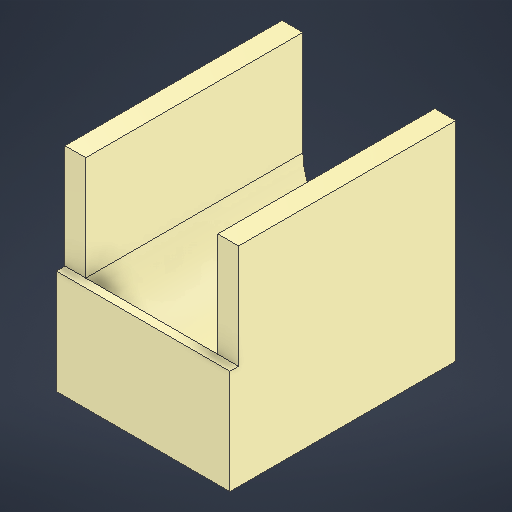
# Autodesk Inventor part: NiMH_Holder_Back
Saved by Autodesk Inventor 2026 (Build 300175050, 175E)
## iProperties
Created: 2025-06-11
Part Number: NiMH_Holder_Back
Material: Generic
Document SubType Name: Modeling
Designer: satom
Density: 1 g/cm^3
Appearance: Default
Author: satom
Autodesk Inventor part; units mm, degrees
ref_plane "YZ Plane" through (0, 0, 0) normal (1, 0, 0) x (0, 1, 0)
ref_plane "XZ Plane" through (0, 0, 0) normal (0, 1, 0) x (-1, 0, 0)
ref_plane "XY Plane" through (0, 0, 0) normal (0, 0, 1) x (1, 0, 0)
sketch "Sketch1" plane through (0, 0, 0) normal (0, 0, 1) x (1, 0, 0)
  line L0 (-15.875, 0) -> (15.875, 0)
  line L1 (15.875, 0) -> (15.875, 38.1)
  line L2 (15.875, 38.1) -> (-15.875, 38.1)
  line L3 (-15.875, 38.1) -> (-15.875, 0)
  point P0 (0, 0)
  dimension "d2" = 31.75
  dimension "d3" = 38.1
  dimension "d4" = 15.875
  dimension "d5" = 0
  constraints: 8 end point, 2 parallel, 1 horizontal, 1 perpendicular
  measures "d2" distance of L0.start L0.end
  measures "d3" distance of L0.end L1.end
  measures "d4" distance from line of point (0, 0) L3
  measures "d5" distance from line of point (0, 0) L0
extrude "Extrusion1" add sketch "Sketch1" along normal blind 139.7
sketch "Sketch2" plane through (0, 0, 139.7) normal (0, 0, 1) x (1, 0, 0)
  arc A0 (-12.065, 19.05) -> (12.065, 19.05) centre (0, 19.05) ccw
  line L0 (-15.875, 0) -> (15.875, 0) projected
  line L1 (12.065, 19.05) -> (12.065, 38.1)
  line L2 (15.875, 38.1) -> (-15.875, 38.1) projected
  line L3 (-12.065, 19.05) -> (-12.065, 38.1)
  point P0 (0, 0)
  dimension "d8" = 19.05
  dimension "d9" = 24.13
  constraints: 4 end point, 2 point on circle, 2 point on line, 1 centre point, 1 parallel, 1 tangent, 1 vertical
  measures "d8" distance from line of L0 A0.centre
  measures "d9" diameter of A0
extrude "Extrusion2" cut sketch "Sketch2" against normal through all
sketch "Sketch3" plane through (-15.875, 0, 0) normal (0, -1, 0) x (1, 0, 0)
  circle A0 centre (28.575, 8.89) radius 2
  circle A1 centre (3.175, 130.81) radius 2
  line L0 (15.875, 0) -> (15.875, 139.7) construction
  line L1 (0, 139.7) -> (31.75, 139.7) construction
  line L2 (0, 0) -> (31.75, 0) construction
  line L3 (31.75, 139.7) -> (0, 139.7) construction
  circle A2 centre (28.575, 111.76) radius 2
  line L4 (31.75, 0) -> (31.75, 139.7) projected
  dimension "d12" = 4
  dimension "d13" = 4
  dimension "d14" = 12.7
  dimension "d15" = 8.89
  dimension "d16" = 12.7
  dimension "d17" = 8.89
  dimension "d28" = 4
  dimension "d30" = 27.94
  dimension "d32" = 12.7
  constraints: 4 end point, 3 centre point, 2 midpoint, 1 collinear
  measures "d12" diameter of A0
  measures "d13" diameter of A1
  measures "d14" distance from line of L0 A0.centre
  measures "d15" distance from line of L2 A0.centre
  measures "d16" distance from line of L0 A1.centre
  measures "d17" vertical distance of L1.start A1.centre
  measures "d28" diameter of A2
  measures "d30" vertical distance of point (15.875, 139.7) A2.centre
  measures "d32" distance from line of A2.centre L0
extrude "Heat Set Inserts" cut sketch "Sketch3" against normal blind 7
sketch "Sketch4" plane through (0, 0, 139.7) normal (0, 0, 1) x (1, 0, 0)
  line L0 (-15.875, 0) -> (15.875, 0) projected
  line L1 (15.875, 0) -> (15.875, 38.1) projected
  line L2 (-15.875, 0) -> (15.875, 0)
  line L3 (15.875, 0) -> (15.875, 19.05)
  line L4 (15.875, 19.05) -> (-15.875, 19.05)
  line L5 (-15.875, 19.05) -> (-15.875, 0)
  point P0 (0, 0)
  dimension "d20" = 19.05
  constraints: 8 end point, 2 parallel, 1 horizontal, 1 midpoint, 1 perpendicular
  measures "d20" distance of L4.end L0.start
extrude "Back Wall" add sketch "Sketch4" along normal blind 1.5875
sketch "Sketch5" plane through (0, 0, 0) normal (0, 0, -1) x (-1, 0, 0)
  line L0 (15.875, 0) -> (-15.875, 0) projected
  line L1 (15.875, 19.05) -> (15.875, 0) projected
  line L2 (-15.875, 0) -> (15.875, 0)
  line L3 (15.875, 0) -> (15.875, 10.16)
  line L4 (15.875, 10.16) -> (-15.875, 10.16)
  line L5 (-15.875, 10.16) -> (-15.875, 0)
  point P0 (0, 0)
  dimension "d23" = 10.16
  constraints: 8 end point, 2 parallel, 1 horizontal, 1 perpendicular, 1 point on line
  measures "d23" distance of L4.end L0.end
extrude "Extrusion5" add sketch "Sketch5" along normal blind 1.5875
sketch "Sketch6" plane through (0, 0, -1.5875) normal (0, 0, -1) x (-1, 0, 0)
  line L0 (15.875, 0) -> (-15.875, 0) projected
  line L1 (-15.875, 38.1) -> (15.875, 38.1)
  line L2 (15.875, 38.1) -> (15.875, 0)
  line L3 (15.875, 0) -> (-15.875, 0)
  line L4 (-15.875, 0) -> (-15.875, 38.1)
  point P0 (0, 0)
  constraints: 8 end point, 2 parallel, 1 horizontal, 1 perpendicular
extrude "Extrusion6" cut sketch "Sketch6" against normal blind 101.6
equation "\"d4\" = 0.5 * d2"
equation "\"d12\" = m3_heat_set_insert"
equation "\"d13\" = m3_heat_set_insert"
equation "\"d28\" = d29"
equation "\"d32\" = d16"
equation "\"d18\" = m3_heat_set_depth"
equation "\"m3_heat_set_insert\" = 4"
equation "\"m3_clearance\" = 3.4"
equation "\"m3_heat_set_depth\" = 7"
equation "\"robot_diameter\" = 354"
equation "\"hardboard_thickness\" = 5"
equation "\"d29\" = 4"
body "Solid1"
